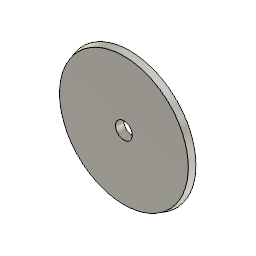
Engrane pequeño 2 v8 (Autodesk Fusion 360 archive; units mm, degrees)
design "Anillo de engrane 2"
Autodesk Fusion 360 part; units mm, degrees
sketch "Boceto1" plane through (0, 0, 0) normal (0, 0, 1) x (1, 0, 0)
  line L0 (0, 0) -> (17.25, 0)
  line L1 (17.25, 0) -> (17.7374, 1.5868)
  line L2 (17.7374, 1.5868) -> (15.6725, 2.221)
  line L3 (15.6725, 2.221) -> (0, 2.221)
  line L4 (0, 2.221) -> (0, 0)
  line L5 (0, 1.5868) -> (17.7374, 1.5868) construction
  dimension "d1" = 17.25
  dimension "d3" = 1.66
  dimension "d4" = 2.16
  dimension "d16" = 90
  dimension "d22" = 2.221
  constraint coincident L0.start L4.end
  constraint horizontal L0
  constraint parallel L0 L3
  constraint perpendicular L0 L4
  constraint coincident L4 L5.start
  constraint perpendicular L4 L5
  measures "d1" distance of L0.start L0.end
  measures "d3" distance of L0.end L1.end
  measures "d4" distance of L1.end L2.end
  measures "d16" angle of L1 L2
  measures "d22" distance of L0 L3
revolve "Revolución2" add sketch "Boceto1" angle 360 about axis through (0, 2.221, 0) along (0, -1, 0)
sketch "Boceto4" plane through (0, 0, 0) normal (0, -1, 0) x (1, 0, 0)
  circle A0 centre (0, 0) radius 17.25
  circle A1 centre (0, 0) radius 2.25
  dimension "d19" = 4.5
  constraint coincident A0.centre A1.centre
  measures "d19" diameter of A1
extrude "Extruir3" cut sketch "Boceto4" along normal mid plane 26 contours A1
